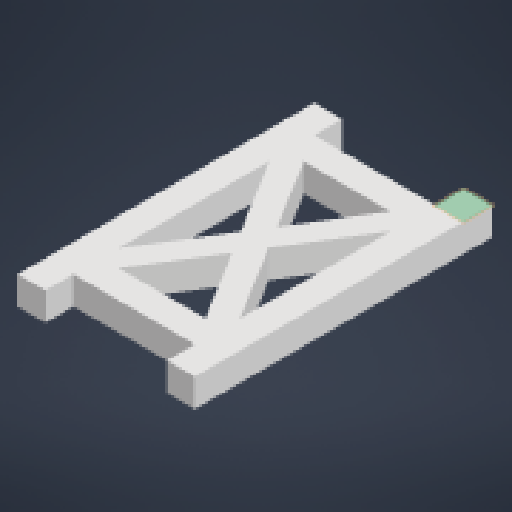
# Autodesk Inventor part: CrossReinforcementUpper
Saved by Autodesk Inventor 2027 (Build 310192000, 192)
## iProperties
Created: 2026-04-15
Part Number: CrossReinforcementUpper
Material: Generic
Document SubType Name: Modeling
Designer: Tueha
Density: 1 g/cm^3
Appearance: Default
Author: Tueha
Autodesk Inventor part; units mm, degrees
ref_plane "YZ Plane" through (0, 0, 0) normal (1, 0, 0) x (0, 1, 0)
ref_plane "XZ Plane" through (0, 0, 0) normal (0, 1, 0) x (-1, 0, 0)
ref_plane "XY Plane" through (0, 0, 0) normal (0, 0, 1) x (1, 0, 0)
ref_plane "Work Plane2" through (-47, 12, 0) normal (0, -1, 0) x (0, 0, -1)
sketch "Sketch2" plane through (-47, 12, 0) normal (0, -1, 0) x (0, 0, -1)
  line L0 (0, 0) -> (0, 6) projected
  line L1 (0, 0) -> (6, 0) projected
  line L2 (6, 6) -> (6, 0) projected
  line L3 (0, 6) -> (6, 6) projected
  line L4 (0, -32) -> (0, -26) projected
  line L5 (0, -32) -> (6, -32) projected
  line L6 (6, -26) -> (6, -32) projected
  line L7 (0, -26) -> (6, -26) projected
  line L8 (-57.6, -32) -> (-57.6, -26) projected
  line L9 (-57.6, -32) -> (-51.6, -32) projected
  line L10 (-51.6, -26) -> (-51.6, -32) projected
  line L11 (-57.6, -26) -> (-51.6, -26) projected
  line L12 (-57.6, 0) -> (-57.6, 6) projected
  line L13 (-57.6, 0) -> (-51.6, 0) projected
  line L14 (-51.6, 6) -> (-51.6, 0) projected
  line L15 (-57.6, 6) -> (-51.6, 6) projected
  line L16 (-51.6, 6) -> (0, 6)
  line L17 (0, 0) -> (-51.6, 0)
  line L18 (-51.6, 0) -> (0, -32)
  line L19 (0, -26) -> (-51.6, 6)
  line L20 (-51.6, -32) -> (0, 0)
  line L21 (-51.6, -26) -> (0, 6)
  line L22 (0, -32) -> (-51.6, -32)
  line L23 (-51.6, -26) -> (0, -26)
  line L24 (-6, 0) -> (-6, -26)
  line L25 (0, 0) -> (0, -26)
  line L26 (-45.6, -26) -> (-45.6, 0)
  line L27 (-51.6, 0) -> (-51.6, -26)
  point P0 (0, 47)
  point P1 (-20.9625, -13)
  point P2 (-6, -3.7209)
  point P3 (-6, -22.2791)
  point P4 (-25.8, -10)
  point P5 (-41.925, 0)
  point P6 (-9.675, 0)
  point P7 (-25.8, -16)
  point P8 (-9.675, -26)
  point P9 (-41.925, -26)
  point P10 (-30.6375, -13)
  point P11 (-45.6, -22.2791)
  point P12 (-45.6, -3.7209)
  constraints: 24 end point, 7 parallel, 4 point on line, 2 perpendicular, 1 horizontal
extrude "Extrusion1" add sketch "Sketch2" along normal blind 6 contours L17 L21 L0 | L0 L3 L2 L1 | L20 L24 L17 | L25 L19 L24 L20 | L21 L17 L19 L16 | L24 L20 L19 L21 L17 | L7 L6 L5 L4 | L23 L24 L19 | L4 L18 L23 | L19 L17 L14 | L14 L13 L12 L15 | L20 L18 L21 L19 | L19 L24 L23 L18 L20 | L22 L20 L23 L18 | L17 L26 L18 | L18 L26 L21 L27 | L19 L21 L18 L26 L17 | L20 L23 L26 L21 L18 | L9 L8 L11 L10 | L10 L23 L20 | L21 L26 L23
body "Solid1"
